Autodesk Inventor part; units mm, degrees
(part 2 of 2)
sketch "Sketch16" plane through (33, 0, 0) normal (-1, 0, 0) x (0, 0, 1)
  line L0 (43.6973, -20.739) -> (43.6973, -19.739) projected
  line L1 (37.4473, -19.739) -> (43.6973, -19.739) projected
  line L2 (37.4473, -18.239) -> (37.4473, -19.739) projected
  line L3 (35.4473, -18.239) -> (37.4473, -18.239) projected
  line L4 (35.4473, -19.739) -> (35.4473, -18.239) projected
  line L5 (33.4473, -19.739) -> (35.4473, -19.739) projected
  line L6 (33.4473, -20.739) -> (33.4473, -19.739) projected
  line L7 (43.6973, -20.739) -> (33.4473, -20.739) projected
  line L8 (58.6973, -19.739) -> (58.6973, -20.739) projected
  line L9 (74.4473, -20.739) -> (58.6973, -20.739) projected
  line L10 (74.4473, -18.239) -> (74.4473, -20.739) projected
  line L11 (64.4473, -18.239) -> (74.4473, -18.239) projected
  line L12 (64.4473, -19.739) -> (64.4473, -18.239) projected
  line L13 (58.6973, -19.739) -> (64.4473, -19.739) projected
  line L14 (43.6973, -20.739) -> (43.6973, -19.739) projected
  line L15 (56.6973, -19.739) -> (58.6973, -19.739) projected
  line L16 (43.6973, -20.739) -> (58.6973, -20.739)
  line L17 (58.6973, -20.739) -> (58.6973, -19.739)
  line L18 (58.6973, -19.739) -> (43.6973, -19.739)
  line L19 (43.6973, -19.739) -> (43.6973, -20.739)
  line L20 (74.4473, -20.739) -> (33.4473, -20.739) projected
  line L21 (35.4473, -20.739) -> (35.4473, -19.739)
  line L22 (64.4473, -18.239) -> (74.4473, -18.239) projected
  line L23 (66.5723, -18.239) -> (66.5723, -20.739)
  point P0 (0, 0)
  constraints: 12 end point, 2 parallel, 2 perpendicular, 2 point on line, 1 horizontal, 1 midpoint
extrude "Extrusion15" add sketch "Sketch16" along normal blind 8 contours L7 L21 L4 L3 L2 L1 L0 | L0 L18 L15 L8 L16 | L8 L13 L12 L11 L23 L9
sketch "Sketch17" plane through (27, -12.299, 69.5623) normal (0, 1, 0) x (1, 0, 0)
  circle A0 centre (37.7, 18.365) radius 3.0166 projected
  arc A1 (30.8, 14.3947) -> (33.7, 11.4947) centre (33.7, 14.3947) ccw projected
  arc A2 (33.7, 25.2947) -> (30.8, 22.3947) centre (33.7, 22.3947) ccw projected
  arc A3 (44.6, 22.3947) -> (41.7, 25.2947) centre (41.7, 22.3947) ccw projected
  arc A4 (41.7, 11.4947) -> (44.6, 14.3947) centre (41.7, 14.3947) ccw projected
  line L0 (52.7389, 29.7327) -> (26.9807, 29.7327)
  line L1 (21.9807, 24.7327) -> (21.9807, 11.7971)
  line L2 (26.9807, 6.7971) -> (52.7389, 6.7971)
  line L3 (57.7389, 11.7971) -> (57.7389, 24.7327)
  arc A5 (52.7389, 6.7971) -> (57.7389, 11.7971) centre (52.7389, 11.7971) ccw
  arc A6 (21.9807, 11.7971) -> (26.9807, 6.7971) centre (26.9807, 11.7971) ccw
  arc A7 (26.9807, 29.7327) -> (21.9807, 24.7327) centre (26.9807, 24.7327) ccw
  arc A8 (57.7389, 24.7327) -> (52.7389, 29.7327) centre (52.7389, 24.7327) ccw
  point P0 (-27, 69.5623)
  dimension "d122" = 5
  constraints: 8 end point, 8 point on circle, 8 tangent, 4 centre point, 3 equal radius, 2 parallel, 1 horizontal, 1 perpendicular
  measures "d122" radius of A5
extrude "Extrusion16" cut sketch "Sketch17" against normal blind 1
sketch "Sketch18" plane through (64.7, -12.299, 51.1973) normal (0, 1, 0) x (1, 0, 0)
  line L0 (-4.865, 4.365) -> (-4.865, -4.365) projected
  line L1 (4.365, 4.865) -> (-4.365, 4.865) projected
  line L2 (-4.365, -4.865) -> (4.365, -4.865) projected
  line L3 (4.865, -4.365) -> (4.865, 4.365) projected
  circle A0 centre (0, 0) radius 3.0166 projected
  circle A1 centre (0, 0) radius 4.05
  point P0 (-64.7, 51.1973)
  dimension "d125" = 8.1
  constraints: 1 centre point, 1 coincident
  measures "d125" diameter of A1
ref_plane "Work Plane4" through (7.664, -19.539, 38.4473) normal (0, -1, 0) x (1, 0, 0)
extrude "Extrusion17" cut sketch "Sketch18" against normal up to surface (7.24 mm away) contours A0 | A1
sketch "Sketch19" plane through (27, -32.299, 69.5623) normal (0, -1, 0) x (1, 0, 0)
  circle A0 centre (37.7, -18.365) radius 3.0166 projected
  circle A1 centre (37.7, -18.365) radius 2.5
  point P0 (-27, -69.5623)
  dimension "d128" = 5
  constraints: 1 centre point, 1 coincident
  measures "d128" diameter of A1
extrude "Extrusion18" cut sketch "Sketch19" against normal up to surface (11.56 mm away) contours A1
sketch "Sketch20" plane through (27, -32.299, 69.5623) normal (0, -1, 0) x (1, 0, 0)
  circle A0 centre (37.7, -18.365) radius 2.5 projected
  circle A1 centre (37.7, -18.365) radius 3.7095
  circle A2 centre (37.7, -18.365) radius 4.05 projected
  line L0 (35.7456, -14.8178) -> (39.2418, -14.8178)
  line L1 (39.2418, -14.8178) -> (39.2418, 2.5656)
  line L2 (39.2418, 2.5656) -> (35.7456, 2.5656)
  line L3 (35.7456, 2.5656) -> (35.7456, -14.8178)
  point P0 (-27, -69.5623)
  constraints: 8 end point, 2 parallel, 1 centre point, 1 coincident, 1 horizontal, 1 perpendicular, 2 other
extrude "Extrusion19" cut sketch "Sketch20" against normal blind 1 contours A0 | A1 L0 | A1 L0 L1 A2 | L0 A1 | A1 L0 A2 L1 | L3 L2 L1 A2
sketch "Sketch21" plane through (27, -12.299, 69.5623) normal (0, 1, 0) x (1, 0, 0)
  circle A0 centre (35, 2.1066) radius 1.45 projected
  line L0 (0, -0.75) -> (70, -0.75) projected
  line L1 (24.0722, -0.75) -> (45.9278, -0.75)
  line L2 (45.9278, -0.75) -> (39.3301, -12.1776)
  line L3 (30.6699, -12.1776) -> (24.0722, -0.75)
  arc A1 (30.6699, -12.1776) -> (39.3301, -12.1776) centre (35, -9.6776) ccw
  circle A2 centre (35, -10.9563) radius 1.45
  point P0 (-27, 69.5623)
  point P1 (35, -7.0592)
  point P2 (35, -19.6776)
  dimension "d133" = 0
  dimension "d134" = 5
  dimension "d135" = 2.9
  constraints: 6 end point, 3 point on line, 2 centre point, 2 point on circle, 2 tangent, 1 collinear, 7 other
  measures "d133" horizontal distance of A0.centre point (35, -7.059)
  measures "d134" radius of A1
  measures "d135" diameter of A2
extrude "Extrusion20" add sketch "Sketch21" against normal up to surface (3.94 mm away) contours L0 L2 A1 L3
sketch "Sketch22" plane through (82, -18.239, 74.4473) normal (0, 1, 0) x (1, 0, 0)
  circle A0 centre (-20, -6.0713) radius 1.45 projected
  line L0 (-30.9278, 4.135) -> (-9.0722, 4.135) projected
  line L1 (-24.3301, -7.2926) -> (-30.9278, 4.135) projected
  arc A1 (-24.3301, -7.2926) -> (-15.6699, -7.2926) centre (-20, -4.7926) ccw projected
  line L2 (-9.0722, 4.135) -> (-15.6699, -7.2926) projected
  line L3 (-24.3301, -7.2926) -> (-30.9278, 4.135) projected
  line L4 (-28.6603, 0.2074) -> (-11.3397, 0.2074)
  point P0 (-82, 74.4473)
  constraints: 2 end point, 2 point on line, 1 horizontal
extrude "Extrusion21" add sketch "Sketch22" against normal up to surface (2.5 mm away) contours A0 | L4 L2 A1 L1
body "Solid1"
